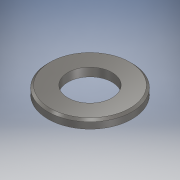
# Autodesk Inventor part: HPCW-M10-A4
Saved by Autodesk Inventor 2019 (Build 230136000, 136)
## iProperties
Created: 2018-04-22
Part Number: HPCW-M10-A4
Material: Stainless Steel AISI 317
Document SubType Name: Modeling
Designer: IEUser
Density: 8 g/cm^3
Appearance: Semi-Polished
Author: IEUser
Autodesk Inventor part; units mm, degrees
ref_plane "YZ Plane" through (0, 0, 0) normal (1, 0, 0) x (0, 1, 0)
ref_plane "XZ Plane" through (0, 0, 0) normal (0, 1, 0) x (-1, 0, 0)
ref_plane "XY Plane" through (0, 0, 0) normal (0, 0, 1) x (1, 0, 0)
sketch "Sketch1" plane through (0, 0, 0) normal (0, 1, 0) x (-1, 0, 0)
  circle A0 centre (0, 0) radius 10
  circle A1 centre (0, 0) radius 5.25
  dimension "d0" = 10.5
  dimension "d1" = 20
  constraints: 2 centre point, 2 coincident
  measures "d0" diameter of A1
  measures "d1" diameter of A0
extrude "Extrusion1" add sketch "Sketch1" along normal blind 2
chamfer "Chamfer1" distance 0.5 angle 45 1 edges at (10, 2, 0)
body "Solid1"
